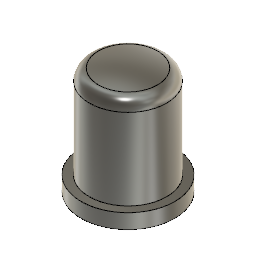
button (Autodesk Fusion 360 design; units mm, degrees)
Autodesk Fusion 360 part; units mm, degrees
note: some values were not read from the file. Set by a fixed rule: which sketch regions a step uses.
sketch "Skizze1" plane through (0, 0, 0) normal (0, 1, 0) x (1, 0, 0)
  line L0 (0, 0) -> (0, -6.7)
  line L1 (0, -6.7) -> (2.35, -6.7)
  line L2 (2.35, -6.7) -> (2.35, -0.9)
  line L3 (2.35, -0.9) -> (2.85, -0.9)
  arc A0 (1.7957, -6.5153) -> (2.35, -5.8339) centre (1.654, -5.8339) ccw
  arc A1 (0, -6.7) -> (1.7957, -6.5153) centre (0, 2.1204) ccw
  line L4 (2.85, -0.9) -> (2.85, 0)
  line L5 (2.85, 0) -> (0, 0)
  dimension "d1" = 2.35
  dimension "d2" = 2.85
  dimension "d9" = 0.1847
  dimension "d10" = 0.5543
  dimension "d13" = 0.9
  dimension "d14" = 6.7
  constraint coincident L0.start L5.end
  constraint vertical L0
  constraint coincident L0 L1.start
  constraint perpendicular L0 L1
  constraint perpendicular L1 L2
  constraint perpendicular L2 L3
  constraint tangent L2 A0
  constraint coincident L2 A0.end
  constraint tangent L1 A1
  constraint tangent A0 A1
  constraint perpendicular L3 L4
  constraint coincident L0 L5.end
  constraint perpendicular L0 L5
  measures "d1" distance of L0.end L1.end
  measures "d2" distance of L0 L3.end
  measures "d9" distance of L1 A0.start
  measures "d10" distance of L2 A0.start
  measures "d13" distance of L3.end L4.end
  measures "d14" distance of L0.start L0.end
revolve "Drehen1" add sketch "Skizze1" angle 360 about axis through (0, 0, 0) along (0, 0, 1) contours L0 L2 L3 A0 A1 L4 L5
equation "d1 = ( 4.7 / 2 ) * 1 mm"
equation "d2 = ( 5.7 / 2 ) * 1 mm"
equation "d14 = 1 mm + 3.5 mm + 0.2 mm + 2 mm"
